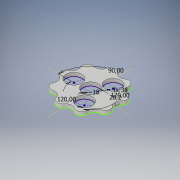
# Autodesk Inventor part: Excenter
Saved by Autodesk Inventor 2018.3 (Build 223284000, 284)
## iProperties
Created: 2018-07-20
Part Number: Excenter
Material: Generisch
Document SubType Name: Modeling
Designer: JochenAlt
Density: 1 g/cm^3
Appearance: Vorgabe
Author: JochenAlt
Autodesk Inventor part; units mm, degrees
ref_plane "YZ Plane" through (0, 0, 0) normal (1, 0, 0) x (0, 1, 0)
ref_plane "XZ Plane" through (0, 0, 0) normal (0, 1, 0) x (-1, 0, 0)
ref_plane "XY Plane" through (0, 0, 0) normal (0, 0, 1) x (1, 0, 0)
sketch "Skizze1" plane through (0, 0, 0) normal (0, 0, 1) x (1, 0, 0)
  line L0 (0, 49.0648) -> (0, -49.0648) construction
  line L1 (-48.0223, 0) -> (46.8814, 0) construction
  circle A0 centre (0, 0) radius 9
  line L2 (0, 0) -> (13.712, 23.7499) construction
  line L3 (0, 0) -> (13.4288, -23.2594) construction
  circle A1 centre (9.5, 16.4545) radius 9
  circle A2 centre (9.5, -16.4545) radius 9
  circle A3 centre (-19, 0) radius 9
  circle A4 centre (0, 0) radius 19 construction
  spline S0 degree 5 poles (28.2, 0) (28.2013, -1.3491) (28.4897, -2.5208) (29.0457, -3.9179) (30.0655, -5.0067) (31.1319, -6.1503) (31.277, -6.3401) (31.6037, -6.8232) (31.8377, -7.3679) (31.9464, -7.6908) (32.1408, -8.4957) (32.1881, -9.3138) (32.1693, -9.7959) (32.0409, -10.7776) (31.7308, -11.7254) (31.5254, -12.1961) (31.0578, -13.0366) (30.4491, -13.7701) (30.1344, -14.0874) (29.5723, -14.555) (28.9286, -14.9219) (28.6661, -15.0434) (28.0946, -15.2554) (27.4982, -15.3452) (27.1938, -15.3745) (24.9338, -15.6332) (22.7968, -16.4501) (21.1967, -17.9941) (20.0139, -20.3053) (19.8068, -22.8891) (19.803, -23.4722) (19.9154, -24.3279) (19.8705, -25.1689) (19.8289, -25.4228) (19.6868, -26.0495) (19.4292, -26.6525) (19.2427, -26.9989) (18.748, -27.7527) (18.1262, -28.4012) (17.7438, -28.7306) (16.9233, -29.312) (16.0096, -29.7319) (15.5331, -29.8984) (14.6605, -30.1125) (13.7604, -30.1642) (13.3672, -30.1524) (12.7162, -30.074) (12.1023, -29.8837) (11.8617, -29.7928) (11.1108, -29.4112) (10.4261, -28.886) (9.9191, -28.5978) (7.5779, -27.4852) (4.985, -27.3539) (2.8478, -27.9677) (1.0718, -29.4099) (-0.2822, -31.2378) (-0.4598, -31.4868) (-0.8358, -31.9583) (-1.3051, -32.3472) (-1.5416, -32.5139) (-2.1812, -32.8879) (-2.867, -33.1409) (-3.2994, -33.2547) (-4.2387, -33.4152) (-5.2007, -33.3998) (-5.7106, -33.3425) (-6.6874, -33.1367) (-7.6005, -32.7577) (-8.0291, -32.5319) (-8.7113, -32.0837) (-9.3142, -31.5107) (-9.5357, -31.2583) (-9.8959, -30.7784) (-10.1454, -30.2589) (-10.2422, -30.0342) (-10.6855, -28.5492) (-11.1602, -27.0906) (-12.0018, -25.9774) (-13.9496, -24.1614) (-16.4961, -23.3826) (-17.881, -23.2103) (-19.3816, -23.5285) (-20.8893, -23.8871) (-21.1322, -23.9156) (-21.7069, -23.9593) (-22.3026, -23.8873) (-22.6319, -23.8216) (-23.4297, -23.586) (-24.1589, -23.2194) (-24.5688, -22.9611) (-25.3535, -22.3598) (-26.0202, -21.6167) (-26.3247, -21.2039) (-26.8191, -20.3784) (-27.1497, -19.4847) (-27.2673, -19.0534) (-27.3911, -18.3329) (-27.387, -17.592) (-27.361, -17.3039) (-27.2588, -16.703) (-27.0384, -16.1416) (-26.9116, -15.8632) (-26.0056, -13.7767) (-25.6446, -11.5175) (-26.1817, -9.3598) (-27.5918, -7.1799) (-29.726, -5.7087) (-30.229, -5.4138) (-31.0263, -5.0833) (-31.7322, -4.6239) (-31.9312, -4.461) (-32.4029, -4.0245) (-32.7964, -3.4999) (-33.0031, -3.1652) (-33.4085, -2.3599) (-33.6593, -1.4972) (-33.7534, -1.0013) (-33.8466, 0) (-33.7534, 1.0013) (-33.6593, 1.4972) (-33.4085, 2.3599) (-33.0031, 3.1652) (-32.7964, 3.4999) (-32.4029, 4.0245) (-31.9312, 4.461) (-31.7322, 4.6239) (-31.0263, 5.0833) (-30.229, 5.4138) (-29.726, 5.7087) (-27.5918, 7.1799) (-26.1817, 9.3598) (-25.6446, 11.5175) (-26.0056, 13.7767) (-26.9116, 15.8632) (-27.0384, 16.1416) (-27.2588, 16.703) (-27.361, 17.3039) (-27.387, 17.592) (-27.3911, 18.3329) (-27.2673, 19.0534) (-27.1497, 19.4847) (-26.8191, 20.3784) (-26.3247, 21.2039) (-26.0202, 21.6167) (-25.3535, 22.3598) (-24.5688, 22.9611) (-24.1589, 23.2194) (-23.4297, 23.586) (-22.6319, 23.8216) (-22.3026, 23.8873) (-21.7069, 23.9593) (-21.1322, 23.9156) (-20.8893, 23.8871) (-19.3816, 23.5285) (-17.881, 23.2103) (-16.4961, 23.3826) (-13.9496, 24.1614) (-12.0018, 25.9774) (-11.1602, 27.0906) (-10.6855, 28.5492) (-10.2422, 30.0342) (-10.1454, 30.2589) (-9.8959, 30.7784) (-9.5357, 31.2583) (-9.3142, 31.5107) (-8.7113, 32.0837) (-8.0291, 32.5319) (-7.6005, 32.7577) (-6.6874, 33.1367) (-5.7106, 33.3425) (-5.2007, 33.3998) (-4.2387, 33.4152) (-3.2994, 33.2547) (-2.867, 33.1409) (-2.1812, 32.8879) (-1.5416, 32.5139) (-1.3051, 32.3472) (-0.8358, 31.9583) (-0.4598, 31.4868) (-0.2822, 31.2378) (1.0718, 29.4099) (2.8478, 27.9677) (4.985, 27.3539) (7.5779, 27.4852) (9.9191, 28.5978) (10.4261, 28.886) (11.1108, 29.4112) (11.8617, 29.7928) (12.1023, 29.8837) (12.7162, 30.074) (13.3672, 30.1524) (13.7604, 30.1642) (14.6605, 30.1125) (15.5331, 29.8984) (16.0096, 29.7319) (16.9233, 29.312) (17.7438, 28.7306) (18.1262, 28.4012) (18.748, 27.7527) (19.2427, 26.9989) (19.4292, 26.6525) (19.6868, 26.0495) (19.8289, 25.4228) (19.8705, 25.1689) (19.9154, 24.3279) (19.803, 23.4722) (19.8068, 22.8891) (20.0139, 20.3053) (21.1967, 17.9941) (22.7968, 16.4501) (24.9338, 15.6332) (27.1938, 15.3745) (27.4982, 15.3452) (28.0946, 15.2554) (28.6661, 15.0434) (28.9286, 14.9219) (29.5723, 14.555) (30.1344, 14.0874) (30.4491, 13.7701) (31.0578, 13.0366) (31.5254, 12.1961) (31.7308, 11.7254) (32.0409, 10.7776) (32.1693, 9.7959) (32.1881, 9.3138) (32.1408, 8.4957) (31.9464, 7.6908) (31.8377, 7.3679) (31.6037, 6.8232) (31.277, 6.3401) (31.1319, 6.1503) (30.0655, 5.0067) (29.0457, 3.9179) (28.4897, 2.5208) (28.2013, 1.3491) (28.2, 0) knots 0 0 0 0 0 0 0.028573 0.028573 0.028573 0.033825 0.033825 0.033825 0.041361 0.041361 0.041361 0.051778 0.051778 0.051778 0.063017 0.063017 0.063017 0.072648 0.072648 0.072648 0.079062 0.079062 0.079062 0.085824 0.085824 0.085824 0.128515 0.128515 0.128515 0.141557 0.141557 0.141557 0.147058 0.147058 0.147058 0.155707 0.155707 0.155707 0.166667 0.166667 0.166667 0.177627 0.177627 0.177627 0.186276 0.186276 0.186276 0.191776 0.191776 0.191776 0.204818 0.204818 0.204818 0.24751 0.24751 0.24751 0.254271 0.254271 0.254271 0.260685 0.260685 0.260685 0.270317 0.270317 0.270317 0.281555 0.281555 0.281555 0.291972 0.291972 0.291972 0.299508 0.299508 0.299508 0.30476 0.30476 0.30476 0.333333 0.333333 0.333333 0.361906 0.361906 0.361906 0.367158 0.367158 0.367158 0.374695 0.374695 0.374695 0.385112 0.385112 0.385112 0.39635 0.39635 0.39635 0.405981 0.405981 0.405981 0.412396 0.412396 0.412396 0.419157 0.419157 0.419157 0.461848 0.461848 0.461848 0.474891 0.474891 0.474891 0.480391 0.480391 0.480391 0.48904 0.48904 0.48904 0.5 0.5 0.5 0.51096 0.51096 0.51096 0.519609 0.519609 0.519609 0.525109 0.525109 0.525109 0.538152 0.538152 0.538152 0.580843 0.580843 0.580843 0.587604 0.587604 0.587604 0.594019 0.594019 0.594019 0.60365 0.60365 0.60365 0.614888 0.614888 0.614888 0.625305 0.625305 0.625305 0.632842 0.632842 0.632842 0.638094 0.638094 0.638094 0.666667 0.666667 0.666667 0.69524 0.69524 0.69524 0.700492 0.700492 0.700492 0.708028 0.708028 0.708028 0.718445 0.718445 0.718445 0.729683 0.729683 0.729683 0.739315 0.739315 0.739315 0.745729 0.745729 0.745729 0.75249 0.75249 0.75249 0.795182 0.795182 0.795182 0.808224 0.808224 0.808224 0.813724 0.813724 0.813724 0.822373 0.822373 0.822373 0.833333 0.833333 0.833333 0.844293 0.844293 0.844293 0.852942 0.852942 0.852942 0.858443 0.858443 0.858443 0.871485 0.871485 0.871485 0.914176 0.914176 0.914176 0.920938 0.920938 0.920938 0.927352 0.927352 0.927352 0.936983 0.936983 0.936983 0.948222 0.948222 0.948222 0.958639 0.958639 0.958639 0.966175 0.966175 0.966175 0.971427 0.971427 0.971427 1 1 1 1 1 1
  line L4 (0, 0) -> (-19, 0) construction
  dimension "d1" = 18
  dimension "d2" = 120
  dimension "d3" = 38
  dimension "d10" = 28.2
  dimension "d11" = 120
  dimension "d12" = 90
  constraints: 6 end point, 5 centre point, 4 point on circle, 4 point on line, 3 equal radius, 1 coincident, 2 other
  measures "d1" diameter of A0
  measures "d2" angle of L2 L3
  measures "d3" diameter of A4
  measures "d10" distance of L2.start point (28.2, 0)
  measures "d11" angle of L3 L4
  measures "d12" angle of L0 L4
extrude "Extrusion1" add sketch "Skizze1" along normal blind 4
equation "curve S0 of \"Skizze1\": x = (38*cos(t))-(7*cos(t+atan(sin(-9*t)/((38/2,8/10)-cos(-9*t)))))-(2,8*cos(10*t)); y = (-38*sin(t))+(7*sin(t+atan(sin(-9*t)/((38/2,8/10)-cos(-9*t)))))+(2,8*sin(10*t)); t from d"
